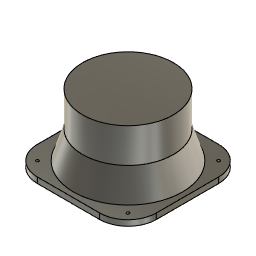
Speaker (Autodesk Fusion 360 design; units mm, degrees)
Autodesk Fusion 360 part; units mm, degrees
sketch "Esquisse1" plane through (0, 0, 0) normal (0, 0, 1) x (1, 0, 0)
  line L0 (27.5, -52.5) -> (-27.5, -52.5)
  line L1 (-52.5, -27.5) -> (-52.5, 27.5)
  line L2 (-27.5, 52.5) -> (27.5, 52.5)
  line L3 (52.5, 27.5) -> (52.5, -27.5)
  circle A0 centre (0, 0) radius 52.5
  line L4 (40, -40) -> (-40, 40) construction
  line L5 (-40, -40) -> (40, 40) construction
  circle A1 centre (-40, -40) radius 1.25
  circle A2 centre (40, -40) radius 1.25
  circle A3 centre (-40, 40) radius 1.25
  circle A4 centre (40, 40) radius 1.25
  arc A5 (-52.5, -27.5) -> (-27.5, -52.5) centre (-27.5, -27.5) ccw
  arc A6 (27.5, -52.5) -> (52.5, -27.5) centre (27.5, -27.5) ccw
  arc A7 (52.5, 27.5) -> (27.5, 52.5) centre (27.5, 27.5) ccw
  arc A8 (-27.5, 52.5) -> (-52.5, 27.5) centre (-27.5, 27.5) ccw
  dimension "d3" = 105
  dimension "d40" = 2.5
  dimension "d41" = 2.5
  dimension "d42" = 2.5
  dimension "d43" = 2.5
  constraint horizontal L0
  constraint perpendicular L0 L1
  constraint parallel L0 L2
  constraint parallel L1 L3
  constraint coincident A0.centre origin
  constraint coincident L4 A0.centre
  constraint coincident L5 A0.centre
  constraint coincident L5.start A1.centre
  constraint coincident L4.start A2.centre
  constraint coincident L4.end A3.centre
  constraint coincident L5.end A4.centre
  constraint tangent L0 A5
  constraint tangent L1 A5
  constraint tangent L0 A6
  constraint tangent L3 A6
  constraint equal A5 A6
  constraint tangent L2 A7
  constraint tangent L3 A7
  constraint equal A5 A7
  constraint tangent L1 A8
  constraint tangent L2 A8
  constraint equal A5 A8
  measures "d3" diameter of A0
  measures "d40" diameter of A1
  measures "d41" diameter of A2
  measures "d42" diameter of A3
  measures "d43" diameter of A4
extrude "Extrusion1" add sketch "Esquisse1" along normal blind 5 contours L0 L3 A0 A6 | L0 L1 A0 A5 | A0 | L1 L2 A0 A8 | L2 L3 A0 A7 | A1 | A2 | A3 | A4
sketch "Esquisse2" plane through (0, 0, 5) normal (0, 0, 1) x (-1, 0, 0)
  line L0 (-27.5, -52.5) -> (27.5, -52.5)
  line L1 (52.5, -27.5) -> (52.5, 27.5)
  line L2 (27.5, 52.5) -> (-27.5, 52.5)
  line L3 (-52.5, 27.5) -> (-52.5, -27.5)
  circle A0 centre (0, 0) radius 48
  arc A1 (-52.5, -27.5) -> (-27.5, -52.5) centre (-27.5, -27.5) ccw
  arc A2 (27.5, -52.5) -> (52.5, -27.5) centre (27.5, -27.5) ccw
  arc A3 (52.5, 27.5) -> (27.5, 52.5) centre (27.5, 27.5) ccw
  arc A4 (-27.5, 52.5) -> (-52.5, 27.5) centre (-27.5, 27.5) ccw
  dimension "d16" = 96
  constraint coincident A0.centre origin
  measures "d16" diameter of A0
extrude "Extrusion2" add sketch "Esquisse2" along normal blind 25 draft -18 contours A0
hole "Perçage2" at (0, 0, 0) direction (0, 0, 1) diameter 80 depth 60 tip angle 180
sketch "Esquisse5" plane through (0, 0, 0) normal (1, 0, 0) x (0, 1, 0)
sketch "Esquisse6" plane through (0, 0, 0) normal (0, 0, 1) x (1, 0, 0)
  circle A0 centre (0, 0) radius 40
  dimension "d28" = 80
  constraint coincident A0.centre origin
  measures "d28" diameter of A0
extrude "Extrusion4" add sketch "Esquisse6" along normal blind 60
hole "Perçage3" at (0, 0, 0) direction (0, 0, 1) diameter 80 depth 5 tip angle 118
extrude "Extrusion6" cut sketch "Esquisse1" along normal blind 5 contours A1 | A2 | A3 | A4
